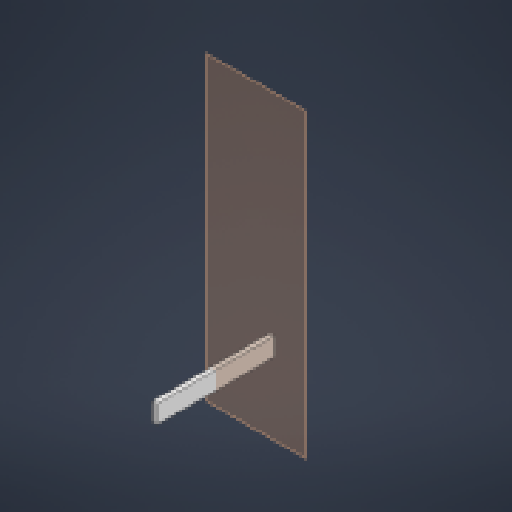
# Autodesk Inventor part: DoorFrameBase
Saved by Autodesk Inventor 2025.1 (Build 291241020, 241B)
## iProperties
Created: 2026-03-06
Part Number: DoorFrameBase
Material: Generic
Document SubType Name: Modeling
Designer: brand
Density: 1 g/cm^3
Appearance: Default
Author: brand
Autodesk Inventor part; units mm, degrees
ref_plane "YZ Plane" through (0, 0, 0) normal (1, 0, 0) x (0, 1, 0)
ref_plane "XZ Plane" through (0, 0, 0) normal (0, 1, 0) x (-1, 0, 0)
ref_plane "XY Plane" through (0, 0, 0) normal (0, 0, 1) x (1, 0, 0)
ref_plane "Work Plane1" through (0, 0, 0) normal (0, 0, 1) x (1, 0, 0)
sketch "Sketch1" plane through (0, 0, 0) normal (0, 0, 1) x (1, 0, 0)
  line L0 (311.15, -1041.4) -> (-311.15, -1041.4) projected
  line L1 (-311.15, -1041.4) -> (-311.15, 1003.3) projected
  line L2 (-311.15, 1003.3) -> (311.15, 1003.3) projected
  line L3 (311.15, 1003.3) -> (311.15, -1041.4) projected
  line L4 (-349.25, 1041.4) -> (-349.25, -1079.5) projected
  line L5 (-349.25, -1079.5) -> (349.25, -1079.5) projected
  line L6 (349.25, -1079.5) -> (349.25, 1041.4) projected
  line L7 (349.25, 1041.4) -> (-349.25, 1041.4) projected
  line L8 (-349.25, -1079.5) -> (-387.35, -1079.5)
  line L9 (-387.35, -1079.5) -> (-387.35, -939.8)
  line L10 (-387.35, -939.8) -> (-349.25, -939.8)
  line L11 (-349.25, -939.8) -> (-349.25, -1079.5)
  point P0 (0, 0)
  dimension "d0" = 38.1
  dimension "d1" = 139.7
  constraints: 8 end point, 2 parallel, 1 horizontal, 1 perpendicular
  measures "d0" distance of L9.end L10.end
  measures "d1" distance of L8.end L9.end
extrude "Extrusion1" add sketch "Sketch1" along normal mid plane 914.4 contours L4 L8 L9 L10
body "Solid1"
